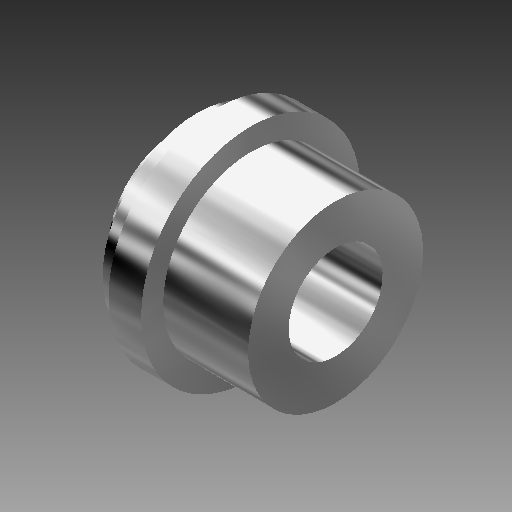
# Autodesk Inventor part: 308-14
Saved by Autodesk Inventor 2019 (Build 230136000, 136)
## iProperties
Company: Autodesk Inc.
Created: 2012-01-24
Part Number: 308-14
Material: Polypropylene
Document SubType Name: Modeling
Designer: Autodesk Inc.
Mass: 0.154726 g
Surface Area: 2.92278 cm^2
Volume: 0.172109 cm^3
Density: 0.899 g/cm^3
Appearance: Chrome - Polished
Author: Inventor
Autodesk Inventor part; units mm, degrees
ref_plane "YZ Plane" through (0, 0, 0) normal (1, 0, 0) x (0, 1, 0)
ref_plane "XZ Plane" through (0, 0, 0) normal (0, 1, 0) x (-1, 0, 0)
ref_plane "XY Plane" through (0, 0, 0) normal (0, 0, 1) x (1, 0, 0)
sketch "Sketch1" plane through (0, 0, 0) normal (0, 0, 1) x (1, 0, 0)
  line L0 (0, 0) -> (0.8, 0)
  line L1 (0.8, 0) -> (0.8, 2.625)
  line L2 (0.8, 2.625) -> (0, 2.625)
  line L3 (0, 2.625) -> (0, 0)
  line L4 (0.8, 0) -> (1.6, 0)
  line L5 (1.6, 0) -> (1.6, 3.625)
  line L6 (1.6, 3.625) -> (0.8, 3.625)
  line L7 (0.8, 3.625) -> (0.8, 0)
  line L8 (1.6, 0) -> (2.85, 0)
  line L9 (2.85, 0) -> (2.85, 4.2)
  line L10 (2.85, 4.2) -> (1.6, 4.2)
  line L11 (1.6, 4.2) -> (1.6, 0)
  line L12 (2.85, 0) -> (6.1, 0)
  line L13 (6.1, 0) -> (6.1, 3.35)
  line L14 (6.1, 3.35) -> (2.85, 3.35)
  line L15 (2.85, 3.35) -> (2.85, 0)
  dimension "d0" = 5.25
  dimension "d1" = 7.25
  dimension "d2" = 8.4
  dimension "d3" = 6.7
  dimension "d4" = 0.8
  dimension "d7" = 1.6
  dimension "d8" = 2.85
  dimension "d9" = 6.1
  constraints: 32 end point, 8 parallel, 4 horizontal, 4 perpendicular
  measures "d0" diameter of L2 L0
  measures "d1" diameter of L6 L0
  measures "d2" diameter of L10 L0
  measures "d3" diameter of L14 L12
  measures "d4" distance of L1.end L2.end
  measures "d7" distance between parallel lines of L3 L11
  measures "d8" distance between parallel lines of L9 L3
  measures "d9" distance between parallel lines of L13 L3
revolve "Revolution1" add sketch "Sketch1" angle 360 about axis through (0, 0, 0) along (1, 0, 0)
hole "Hole1" at (0, 0, 0) direction (1, 0, 0) diameter 3.6 end through all
body "Solid1"
